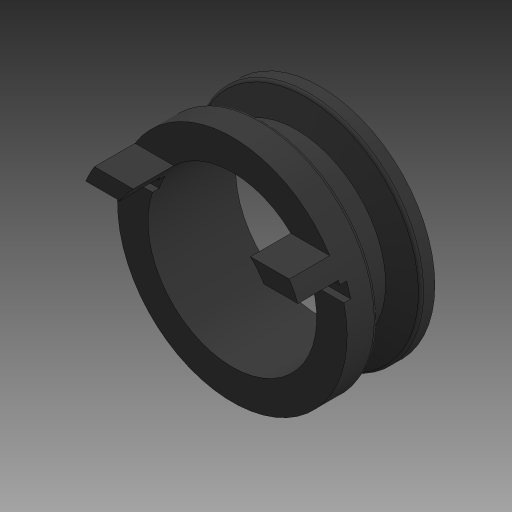
# Autodesk Inventor part: sonar
Saved by Autodesk Inventor 2023 (Build 270158000, 158)
## iProperties
Created: 2024-02-02
Part Number: sonar
Material: Všeobecné
Document SubType Name: Modeling
Designer: matej
Mass: 3.60459 g
Surface Area: 38.9736 cm^2
Volume: 3.60459 cm^3
Density: 1 g/cm^3
Appearance: Guma – černá
Author: matej
Autodesk Inventor part; units mm, degrees
ref_plane "YZ Plane" through (0, 0, 0) normal (1, 0, 0) x (0, 1, 0)
ref_plane "XZ Plane" through (0, 0, 0) normal (0, 1, 0) x (-1, 0, 0)
ref_plane "XY Plane" through (0, 0, 0) normal (0, 0, 1) x (1, 0, 0)
sketch "Náčrt1" plane through (0, 0, 0) normal (0, 0, 1) x (1, 0, 0)
  circle A0 centre (0, 0) radius 17
  circle A1 centre (0, 0) radius 12.5
  line L0 (-2.5, -12.5) -> (2.5, -12.5)
  line L1 (2.5, -12.5) -> (2.5, 12.5)
  line L2 (2.5, 12.5) -> (-2.5, 12.5)
  line L3 (-2.5, 12.5) -> (-2.5, -12.5)
  line L4 (-2.5, -12.5) -> (2.5, 12.5) construction
  line L5 (2.5, -12.5) -> (-2.5, 12.5) construction
  line L6 (-12.5, -2.5) -> (12.5, -2.5)
  line L7 (12.5, -2.5) -> (12.5, 2.5)
  line L8 (12.5, 2.5) -> (-12.5, 2.5)
  line L9 (-12.5, 2.5) -> (-12.5, -2.5)
  line L10 (-12.5, -2.5) -> (12.5, 2.5) construction
  line L11 (12.5, -2.5) -> (-12.5, 2.5) construction
  dimension "d0" = 34
  dimension "d3" = 25
  dimension "d29" = 5
  dimension "d30" = 25
  dimension "d31" = 25
  dimension "d32" = 5
  constraints: 24 end point, 4 midpoint, 4 parallel, 2 centre point, 2 coincident, 2 horizontal, 2 perpendicular
  measures "d0" diameter of A0
  measures "d3" diameter of A1
  measures "d29" distance of L2.end L1.end
  measures "d30" distance of L1.end L0.end
  measures "d31" distance of L8.end L7.end
  measures "d32" distance of L7.end L6.end
extrude "Vysunutí1" add sketch "Náčrt1" along normal blind 13 contours A0 | L7 L6 A1 | A1 L8 L7 | A1 L2 L1 | L1 L0 A1 | A1 L3 L2 | L0 L3 A1 | A1 L9 L8 | L6 L9 A1
sketch "Náčrt2" plane through (0, 0, 0) normal (1, 0, 0) x (0, 1, 0)
  line L0 (17, 0) -> (-17, 0) projected
  circle A0 centre (15, 0) radius 1.1
  line L1 (17, 13) -> (-17, 13) projected
  line L2 (17, 0) -> (-17, 0) projected
  line L3 (-12.5, 13) -> (12.5, 13) projected
  line L4 (-12.5, 0) -> (12.5, 0) projected
  line L5 (17, 0) -> (17, 13) projected
  line L6 (12.5, 13) -> (12.5, 0) projected
  line L7 (0, -3.92) -> (0, 15.82) projected
  point P0 (0, 0)
  point P1 (13.9, 0)
  point P2 (16.1, 0)
  dimension "d4" = 2.2
  dimension "d6" = 2
  dimension "d7" = 2.5
  constraints: 1 centre point, 1 point on line
  measures "d4" diameter of A0
  measures "d6" distance from line of L5 A0.centre
  measures "d7" distance from line of A0.centre L6
revolve "Rotace1" cut sketch "Náčrt2" angle 360 about axis through (0, 0, -10) along (0, 0, 1) picked at (15.2396, 0.5599) contours L0 A0
sketch "Náčrt4" plane through (0, 0, 13) normal (0, 0, 1) x (1, 0, 0)
  line L0 (-17, 6) -> (17, 6)
  line L1 (17, 6) -> (17, 4)
  line L2 (17, 4) -> (-17, 4)
  line L3 (-17, 4) -> (-17, 6)
  line L4 (-17, 6) -> (17, 4) construction
  line L5 (17, 6) -> (-17, 4) construction
  point P0 (0, 0)
  point P1 (0, 5)
  dimension "d9" = 2
  dimension "d10" = 34
  dimension "d11" = 5
  constraints: 12 end point, 2 midpoint, 2 parallel, 1 horizontal, 1 perpendicular, 1 vertical alignment
  measures "d9" distance of L0.end L1.end
  measures "d10" distance of L0.start L0.end
  measures "d11" distance of point (0, 0) point (0, 5)
extrude "Vysunutí2" cut sketch "Náčrt4" against normal blind 1
sketch "Náčrt5" plane through (0, 0, 0) normal (1, 0, 0) x (0, 1, 0)
  line L0 (17, 0) -> (17, 13) projected
  line L1 (17, 2) -> (13.2, 3.5)
  line L2 (17, 2) -> (21.0853, 2) construction
  line L3 (17, 0) -> (-17, 0) projected
  line L4 (13.2, 3.5) -> (13.2, 6.5)
  line L5 (17, 2) -> (17, 8.6939)
  line L6 (17, 8.6939) -> (13.2, 6.5)
  line L7 (0, -2.6) -> (0, 15.6) projected
  point P0 (0, 0)
  point P1 (0, 0)
  dimension "d15" = 2
  dimension "d16" = 13.2
  dimension "d17" = 60
  dimension "d20" = 3.5
  dimension "d21" = 68.459
  dimension "d22" = 3
  constraints: 10 end point, 2 point on line, 1 equal length, 1 horizontal, 1 midpoint, 1 vertical
  measures "d15" distance from line of L3 L1.start
  measures "d16" distance from line of point (0, 0) L4
  measures "d17" angle of L0 L6
  measures "d20" distance from line of L3 L1.end
  measures "d21" angle of L0 L1
  measures "d22" distance of L1.end L4.end
revolve "Rotace2" cut sketch "Náčrt5" angle 360 about axis through (0, 0, -10) along (0, 0, 1)
fillet "Zaoblení1" radius 0.5 4 edges at (12.0208, 12.0208, 8.6939) (-12.0208, -12.0208, 8.6939) (-12.0208, -12.0208, 2) (12.0208, 12.0208, 2)
sketch "Náčrt6" plane through (0, 0, 13) normal (0, 0, 1) x (1, 0, 0)
  circle A0 centre (0, 0) radius 17
  circle A1 centre (0, 0) radius 12.5
  line L0 (17, -9) -> (-17, -9)
  line L1 (-17, -9) -> (-17, 9)
  line L2 (-17, 9) -> (17, 9)
  line L3 (17, 9) -> (17, -9)
  line L4 (17, -9) -> (-17, 9) construction
  line L5 (-17, -9) -> (17, 9) construction
  line L6 (17, -6.5) -> (-17, -6.5)
  line L7 (-17, -6.5) -> (-17, 6.5)
  line L8 (-17, 6.5) -> (17, 6.5)
  line L9 (17, 6.5) -> (17, -6.5)
  line L10 (17, -6.5) -> (-17, 6.5) construction
  line L11 (-17, -6.5) -> (17, 6.5) construction
  point P0 (10.6771, 6.5)
  point P1 (15.7083, 6.5)
  point P2 (14.4222, 9)
  point P3 (8.6747, 9)
  point P4 (-15.7083, 6.5)
  point P5 (-10.6771, 6.5)
  point P6 (-8.6747, 9)
  point P7 (-14.4222, 9)
  dimension "d23" = 34
  dimension "d24" = 13
  dimension "d25" = 34
  dimension "d26" = 18
  constraints: 24 end point, 4 midpoint, 4 parallel, 2 centre point, 2 coincident, 2 horizontal, 2 perpendicular
  measures "d23" distance of L7.end L8.end
  measures "d24" distance of L6.end L7.end
  measures "d25" distance of L1.end L2.end
  measures "d26" distance of L0.end L1.end
extrude "Vysunutí3" add sketch "Náčrt6" along normal blind 6 contours L8 A1 L2 A0 | L2 A1 L8 A0
